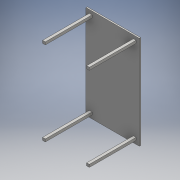
# Autodesk Inventor part: Table
Saved by Autodesk Inventor 2016 SP1 (Build 200210100, 210)
## iProperties
Created: 2016-10-04
Part Number: Table
Material: Générique
Document SubType Name: Modeling
Designer: dimercur
Density: 1 g/cm^3
Appearance: Par défaut
TableLong: 1400,000 mm
Author: dimercur
Autodesk Inventor part; units mm, degrees
ref_plane "YZ Plane" through (0, 0, 0) normal (1, 0, 0) x (0, 1, 0)
ref_plane "XZ Plane" through (0, 0, 0) normal (0, 1, 0) x (-1, 0, 0)
ref_plane "XY Plane" through (0, 0, 0) normal (0, 0, 1) x (1, 0, 0)
sketch "Esquisse1" plane through (0, 0, 0) normal (0, 1, 0) x (-1, 0, 0)
  line L0 (400, 700) -> (-400, 700)
  line L1 (-400, 700) -> (-400, -700)
  line L2 (-400, -700) -> (400, -700)
  line L3 (400, -700) -> (400, 700)
  point P0 (0, 0)
  dimension "TableLong" = 1400
  dimension "TableLarg" = 800
  dimension "d2" = 700
  dimension "d3" = 400
  constraints: 8 end point, 2 parallel, 1 horizontal, 1 perpendicular
  measures "TableLong" distance of L2.end L0.start
  measures "TableLarg" distance of L0.start L0.end
  measures "d2" vertical distance of point (0, 0) L0.start
  measures "d3" horizontal distance of point (0, 0) L0.start
extrude "Extrusion1" add sketch "Esquisse1" along normal blind 20
sketch "Esquisse2" plane through (0, 0, 0) normal (0, -1, 0) x (1, 0, 0)
  line L0 (-400, 700) -> (400, 700) projected
  line L1 (-400, -700) -> (-400, 700) projected
  line L2 (350, 650) -> (310, 650)
  line L3 (310, 650) -> (310, 610)
  line L4 (310, 610) -> (350, 610)
  line L5 (350, 610) -> (350, 650)
  line L6 (400, 700) -> (400, -700) projected
  line L7 (350, -610) -> (310, -610)
  line L8 (310, -610) -> (310, -650)
  line L9 (310, -650) -> (350, -650)
  line L10 (350, -650) -> (350, -610)
  line L11 (-310, 650) -> (-350, 650)
  line L12 (-350, 650) -> (-350, 610)
  line L13 (-350, 610) -> (-310, 610)
  line L14 (-310, 610) -> (-310, 650)
  line L15 (-310, -610) -> (-350, -610)
  line L16 (-350, -610) -> (-350, -650)
  line L17 (-350, -650) -> (-310, -650)
  line L18 (-310, -650) -> (-310, -610)
  point P0 (0, 0)
  dimension "d17" = 50
  dimension "d18" = 50
  dimension "d19" = 40
  dimension "d20" = 40
  dimension "d23" = 1260
  dimension "d30" = 660
  constraints: 32 end point, 2 horizontal, 2 parallel, 1 perpendicular, 1 vertical, 24 other
  measures "d17" distance between parallel lines of L0 L2
  measures "d18" distance between parallel lines of L6 L5
  measures "d19" distance of L2.start L2.end
  measures "d20" distance of L2.end L3.end
  measures "d23" distance of L2.start L7.start
  measures "d30" distance of L2.start L11.start
extrude "Extrusion2" add sketch "Esquisse2" along normal blind 700
equation "\"d2\" = 0.5 * TableLong"
equation "\"d3\" = 0.5 * TableLarg"
equation "\"d23\" = -2 * d17 + TableLong - d20"
equation "\"d30\" = -2 * d18 + TableLarg - d19"
